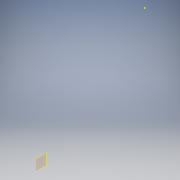
# Autodesk Inventor part: usb Wire
Saved by Autodesk Inventor 2018 (Build 220112000, 112)
## iProperties
Created: 2018-07-20
Part Number: usb Wire
Material: Generic
Document SubType Name: Modeling
Designer: DPLXuser
Density: 1 g/cm^3
Appearance: Default
Author: DPLXuser
Autodesk Inventor part; units mm, degrees
ref_plane "YZ Plane" through (0, 0, 0) normal (1, 0, 0) x (0, 1, 0)
ref_plane "XZ Plane" through (0, 0, 0) normal (0, 1, 0) x (-1, 0, 0)
ref_plane "XY Plane" through (0, 0, 0) normal (0, 0, 1) x (1, 0, 0)
ref_plane "Work Plane1" through (90.6066, -57.8144, 73.5154) normal (1, 0, 0) x (0, 0, 1)
sketch "Sketch1" plane through (90.6066, -57.8144, 73.5154) normal (1, 0, 0) x (0, 0, 1)
  circle A0 centre (0, 0) radius 1.27
  point P0 (-73.5154, -57.8144)
  dimension "d0" = 2.54
  constraints: 1 centre point
  measures "d0" diameter of A0
ref_plane "Work Plane2" through (101.0004, -122.0907, 74.7595) normal (1, 0, 0) x (0, 1, 0)
sketch "Sketch2" plane through (101.0004, -122.0907, 74.7595) normal (1, 0, 0) x (0, 1, 0)
  circle A0 centre (0, 0) radius 3.5687
  point P0 (122.0907, -74.7595)
  dimension "d1" = 7.1374
  constraints: 1 centre point
  measures "d1" diameter of A0
ref_plane "Work Plane3" through (90.6066, -57.8144, 73.5154) normal (0.0901, -0.0047, -0.9959) x (0.1596, -0.987, 0.0191)
sketch "Sketch3" plane through (90.6066, -57.8144, 73.5154) normal (0.0901, -0.0047, -0.9959) x (0.1596, -0.987, 0.0191)
  line L0 (0, 0) -> (9.0654, -45.3035) construction
  line L1 (9.0654, -45.3035) -> (72.5715, -45.3035) construction
  line L2 (72.5715, -45.3035) -> (65.1146, -18.9726) construction
  line L3 (65.1146, -18.9726) -> (65.1146, 0) construction
  spline S0 degree 4 poles (0, 0) (9.0654, -45.3035) (72.5715, -45.3035) (65.1146, -18.9726) (65.1146, 0) knots 1 1 1 1 1 2 2 2 2 2
  point P0 (-72.928, 86.2665)
  constraints: 1 horizontal, 3 other
sweep "Sweep1" add profiles "Sketch1" path "Sketch3"
body "Solid1"
